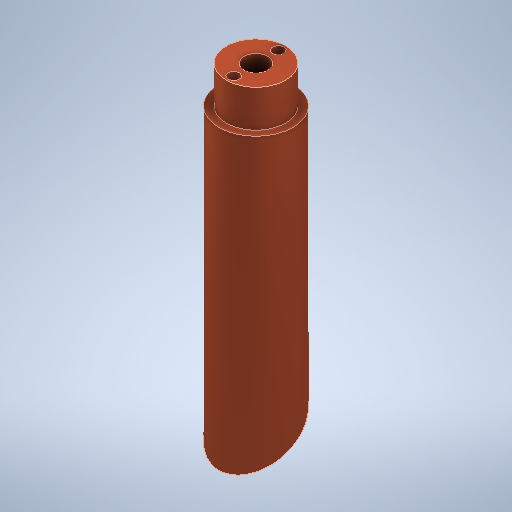
# Autodesk Inventor part: End-tip Coupler
Saved by Autodesk Inventor 2026.2 (Build 302298010, 298A)
## iProperties
Created: 2026-04-29
Part Number: End-tip Coupler
Material: Copper
Document SubType Name: Modeling
Designer: piete
Density: 8.94 g/cm^3
Appearance: Copper - Satin
Author: piete
Autodesk Inventor part; units mm, degrees
ref_plane "YZ Plane" through (0, 0, 0) normal (1, 0, 0) x (0, 1, 0)
ref_plane "XZ Plane" through (0, 0, 0) normal (0, 1, 0) x (-1, 0, 0)
ref_plane "XY Plane" through (0, 0, 0) normal (0, 0, 1) x (1, 0, 0)
sketch "Sketch1" plane through (0, 0, 0) normal (0, 1, 0) x (-1, 0, 0)
  circle A0 centre (0, 0) radius 5
  circle A1 centre (0, 0) radius 1.6
  dimension "d0" = 10
  dimension "d1" = 3.2
  constraints: 2 centre point, 2 coincident
  measures "d0" diameter of A0
  measures "d1" diameter of A1
extrude "Extrusion1" add sketch "Sketch1" along normal blind 45
sketch "Sketch2" plane through (0, 45, 0) normal (0, 1, 0) x (1, 0, 0)
  circle A0 centre (0, 3) radius 0.75
  circle A1 centre (0, -3) radius 0.75
  point P0 (0, 0)
  dimension "d4" = 1.5
  dimension "d5" = 1.5
  dimension "d6" = 6
  dimension "d7" = 3
  dimension "d8" = 0
  dimension "d10" = 0
  constraints: 2 centre point
  measures "d4" diameter of A0
  measures "d5" diameter of A1
  measures "d6" distance of A0.centre A1.centre
  measures "d7" distance of A0.centre point (0, 0)
  measures "d8" horizontal distance of point (0, 0) A1.centre
  measures "d10" horizontal distance of point (0, 0) A0.centre
extrude "Extrusion2" cut sketch "Sketch2" against normal through all
sketch "Sketch3" plane through (0, 0, 0) normal (0, -1, 0) x (1, 0, 0)
  circle A0 centre (0, 0) radius 4.5
  dimension "d13" = 9
  constraints: 1 centre point, 1 coincident
  measures "d13" diameter of A0
extrude "Extrusion3" cut sketch "Sketch3" against normal blind 35
sketch "Sketch4" plane through (0, 0, 0) normal (1, 0, 0) x (0, 1, 0)
  line L0 (0, -5) -> (0, 5) projected
  line L1 (0, 5) -> (5.7735, -5)
  line L2 (0, -5) -> (45, -5) projected
  line L3 (0, 5) -> (11.547, 5) construction
  line L4 (5.7735, -5) -> (0, -5)
  line L5 (0, 5) -> (0, -5)
  point P0 (0, 0)
  dimension "d16" = 60
  constraints: 8 end point, 2 point on line, 1 equal length, 1 horizontal, 1 perpendicular
  measures "d16" angle of L1 L3
extrude "Extrusion4" cut sketch "Sketch4" along normal through all both and the other way through all
sketch "Sketch5" plane through (0, 45, 0) normal (0, 1, 0) x (1, 0, 0)
  circle A0 centre (0, 0) radius 5
  circle A1 centre (0, 0) radius 4
  dimension "d19" = 10
  dimension "d20" = 8
  constraints: 2 centre point, 2 coincident
  measures "d19" diameter of A0
  measures "d20" diameter of A1
extrude "Extrusion5" cut sketch "Sketch5" against normal blind 5
body "Solid1"
